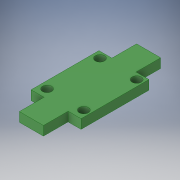
# Autodesk Inventor part: КВ33.044.503 - Прижим ремня
Saved by Autodesk Inventor 2019 (Build 230136000, 136)
## iProperties
Created: 2019-08-04
Part Number: КВ33.044.503 - Прижим ремня
Material: Пластик АБС
Document SubType Name: Modeling
Designer: Петров Иван
Density: 1.06 g/cm^3
Appearance: Гладкий — темный травянисто-зеленый
Author: Петров Иван
Autodesk Inventor part; units mm, degrees
ref_plane "YZ Plane" through (0, 0, 0) normal (1, 0, 0) x (0, 1, 0)
ref_plane "XZ Plane" through (0, 0, 0) normal (0, 1, 0) x (-1, 0, 0)
ref_plane "XY Plane" through (0, 0, 0) normal (0, 0, 1) x (1, 0, 0)
sketch "Эскиз1" plane through (0, 0, 0) normal (0, 1, 0) x (-1, 0, 0)
  circle A0 centre (6.2967, 9.3442) radius 1.5
  circle A1 centre (-5.6093, 9.3442) radius 1.5
  circle A2 centre (-5.6093, -7.7911) radius 1.5
  circle A3 centre (6.2967, -7.7911) radius 1.5
  line L0 (4.4235, -9.7991) -> (4.4235, -17.7991)
  line L1 (8.6235, -9.7991) -> (4.4235, -9.7991)
  line L2 (8.6235, 12.2009) -> (8.6235, -9.7991)
  line L3 (4.4235, 12.2009) -> (8.6235, 12.2009)
  line L4 (4.4235, 20.2009) -> (4.4235, 12.2009)
  line L5 (-3.3765, 20.2009) -> (4.4235, 20.2009)
  line L6 (-3.3765, 12.2009) -> (-3.3765, 20.2009)
  line L7 (-7.5765, 12.2009) -> (-3.3765, 12.2009)
  line L8 (-7.5765, -9.7991) -> (-7.5765, 12.2009)
  line L9 (-3.3765, -9.7991) -> (-7.5765, -9.7991)
  line L10 (-3.3765, -17.7991) -> (-3.3765, -9.7991)
  line L11 (4.4235, -17.7991) -> (-3.3765, -17.7991)
  point P0 (0, 0)
  point P1 (-15.7765, 1.2009)
  constraints: 24 end point, 4 centre point
extrude "Выдавливание1" add sketch "Эскиз1" along normal blind 3
